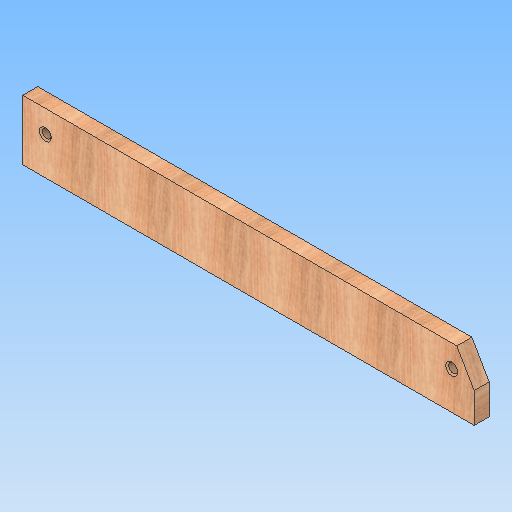
# Autodesk Inventor part: Top_Floor Plank
Saved by Autodesk Inventor 2018.1 (Build 221171000, 171)
## iProperties
Created: 2019-03-15
Part Number: Top_Floor Plank
Material: Wood (Birch)
Document SubType Name: Modeling
Designer: James
Density: 0.55 g/cm^3
Appearance: Birch - Natural Polished
Mass: 8128.86 g
Surface Area: 7677.37 cm^2
Volume: 14779.7 cm^3
Author: James
Autodesk Inventor part; units mm, degrees
ref_plane "YZ Plane" through (0, 0, 0) normal (1, 0, 0) x (0, 1, 0)
ref_plane "XZ Plane" through (0, 0, 0) normal (0, 1, 0) x (-1, 0, 0)
ref_plane "XY Plane" through (0, 0, 0) normal (0, 0, 1) x (1, 0, 0)
sketch "Sketch1" plane through (0, 0, 0) normal (0, 0, 1) x (1, 0, 0)
  line L0 (0, 0) -> (1500, 0)
  line L1 (1500, 0) -> (1500, 200)
  line L2 (1500, 200) -> (0, 200)
  line L3 (0, 200) -> (0, 0)
  dimension "d0" = 200
  dimension "d1" = 1500
  constraints: 8 end point, 2 parallel, 1 horizontal, 1 perpendicular
  measures "d0" distance of L0.end L1.end
  measures "d1" distance of L1.end L2.end
extrude "Extrusion1" add sketch "Sketch1" along normal blind 50
sketch "Sketch2" plane through (0, 0, 50) normal (0, 0, 1) x (1, 0, 0)
  line L0 (0, 200) -> (0, 0) projected
  line L1 (1500, 0) -> (1500, 200) projected
  line L2 (1500, 200) -> (0, 200) projected
  point P0 (75, 125)
  point P1 (1425, 125)
  point P2 (0, 100)
  dimension "d4" = 75
  dimension "d5" = 75
  dimension "d19" = 75
  constraints: 1 horizontal alignment, 1 midpoint
  measures "d4" distance from line of point (75, 125) L0
  measures "d5" distance from line of L1 point (1425, 125)
  measures "d19" distance from line of point (75, 125) L2
hole "Hole1" at (75, 125, 50) at (1425, 125, 50) direction (0, 0, -1) diameter 30 end through all
chamfer "Chamfer1" distance 5 angle 45 4 edges at (75, 140, 50) (1425, 140, 50) (75, 140, 0) (1425, 140, 0)
chamfer "Chamfer2" distance 100 angle 30 1 edges at (1500, 200, 25) measured on face at (1500, 66.6667, 16.6667)
body "Solid1"
